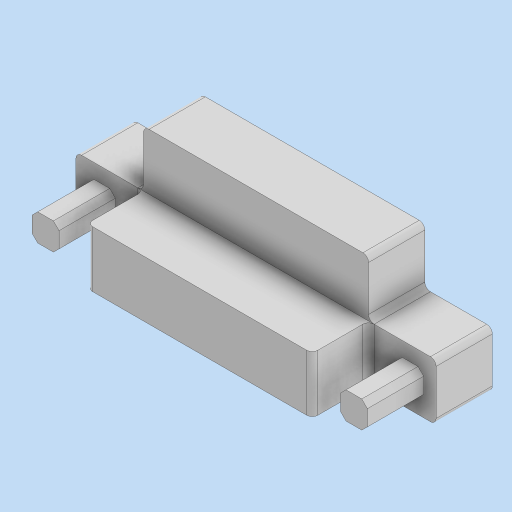
# Autodesk Inventor part: UNION_CHEWIE
Saved by Autodesk Inventor 2024 (Build 280153000, 153)
## iProperties
Created: 2024-11-05
Part Number: UNION_CHEWIE
Material: Generic
Document SubType Name: Modeling
Designer: MxMon
Density: 1 g/cm^3
Appearance: Default
Author: MxMon
Autodesk Inventor part; units mm, degrees
ref_plane "YZ Plane" through (0, 0, 0) normal (1, 0, 0) x (0, 1, 0)
ref_plane "XZ Plane" through (0, 0, 0) normal (0, 1, 0) x (-1, 0, 0)
ref_plane "XY Plane" through (0, 0, 0) normal (0, 0, 1) x (1, 0, 0)
sketch "Sketch1" plane through (0, 0, 0) normal (0, 0, 1) x (1, 0, 0)
  line L0 (-20, 10) -> (20, 10)
  line L1 (20, 10) -> (20, -10)
  line L2 (20, -10) -> (-20, -10)
  line L3 (-20, -10) -> (-20, 10)
  line L4 (-20, 10) -> (20, -10) construction
  line L5 (20, 10) -> (-20, -10) construction
  line L6 (20, -10) -> (32, -10)
  line L7 (32, -10) -> (32, 0)
  line L8 (32, 0) -> (20, 0)
  line L9 (0, 10) -> (0, -10) construction
  line L10 (-20, -10) -> (-32, -10)
  line L11 (-32, -10) -> (-32, 0)
  line L12 (-32, 0) -> (-20, 0)
  point P0 (0, 0)
  dimension "d0" = 40
  dimension "d1" = 20
  dimension "d4" = 12
  constraints: 26 end point, 5 midpoint, 3 parallel, 3 symmetric about line, 2 horizontal, 2 perpendicular
  measures "d0" distance of L1.end L2.end
  measures "d1" distance of L0.end L1.end
  measures "d4" distance of L1.end L6.end
extrude "Extrusion1" add sketch "Sketch1" against normal blind 10
sketch "Sketch2" plane through (0, 0, 0) normal (0, 0, 1) x (1, 0, 0)
  line L0 (-29.8, -2.6) -> (-25, -2.6)
  line L1 (-25, -2.6) -> (-25, -7.4)
  line L2 (-25, -7.4) -> (-29.8, -7.4)
  line L3 (-29.8, -7.4) -> (-29.8, -2.6)
  line L4 (-29.8, -2.6) -> (-25, -7.4) construction
  line L5 (-25, -2.6) -> (-29.8, -7.4) construction
  line L6 (-32, 0) -> (-32, -10) projected
  line L7 (-20, 0) -> (-32, 0) projected
  line L8 (20, 10) -> (-20, 10) construction
  line L9 (-32, -10) -> (32, -10) construction
  line L10 (0, 10) -> (0, -10) construction
  line L11 (29.8, -2.6) -> (25, -2.6)
  line L12 (25, -2.6) -> (25, -7.4)
  line L13 (25, -7.4) -> (29.8, -7.4)
  line L14 (29.8, -7.4) -> (29.8, -2.6)
  point P0 (0, 0)
  point P1 (-27.4, -5)
  point P2 (-32, -5)
  point P3 (-26, 0)
  point P4 (-25, -5)
  dimension "d5" = 4.8
  dimension "d6" = 4.8
  dimension "d12" = 5
  constraints: 22 end point, 7 midpoint, 4 symmetric about line, 2 parallel, 1 horizontal, 1 horizontal alignment, 1 perpendicular
  measures "d5" distance of L1.end L2.end
  measures "d6" distance of L0.end L1.end
  measures "d12" horizontal distance of L7.start point (-25, -5)
extrude "Extrusion2" add sketch "Sketch2" along normal blind 10
chamfer "Chamfer1" distance 1 angle 45 8 edges at (-25, -2.6, 5) (-29.8, -2.6, 5) (-29.8, -7.4, 5) (-25, -7.4, 5) (25, -2.6, 5) (29.8, -2.6, 5) (29.8, -7.4, 5) (25, -7.4, 5)
sketch "Sketch3" plane through (0, 0, 0) normal (0, 0, 1) x (1, 0, 0)
  line L0 (32, -10) -> (-32, -10) projected
  line L1 (20, -10) -> (-20, -10)
  line L2 (-20, -10) -> (-20, 0)
  line L3 (-20, 0) -> (20, 0)
  line L4 (20, 0) -> (20, -10)
  point P0 (0, 0)
  point P1 (-20, 0)
  point P2 (-20, -10)
  dimension "d13" = 40
  constraints: 8 end point, 2 parallel, 1 coincident, 1 horizontal, 1 perpendicular, 1 point on line
  measures "d13" distance of L2.end L3.end
extrude "Extrusion3" add sketch "Sketch3" along normal blind 10
fillet "Fillet1" radius 1 1 edges at (-20, -5, 0)
fillet "Fillet2" radius 1 1 edges at (20, -5, 0)
fillet "Fillet3" radius 1 8 edges at (-32, -10, -5) (32, -10, -5) (32, 0, -5) (20, 10, -5) (-20, 10, -5) (-20, 0, -5) (20, 0, -5) (-32, 0, -5)
fillet "Fillet4" radius 1 2 edges at (-20, -5, 10) (20, -5, 10)
body "Solid1"
